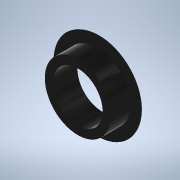
# Autodesk Inventor part: 08-02-01-010_buttonSide
Saved by Autodesk Inventor 2020 (Build 240168000, 168)
## iProperties
Created: 2021-08-25
Part Number: 08-02-01-010_buttonSide
Material: ABS-Kunststoff(1)
Document SubType Name: Modeling
Designer: Eric
Density: 1.06 g/cm^3
Appearance: Glatt - Weiß(1)
Author: Eric
Autodesk Inventor part; units mm, degrees
ref_plane "YZ Plane" through (0, 0, 0) normal (1, 0, 0) x (0, 1, 0)
ref_plane "XZ Plane" through (0, 0, 0) normal (0, 1, 0) x (-1, 0, 0)
ref_plane "XY Plane" through (0, 0, 0) normal (0, 0, 1) x (1, 0, 0)
sketch "Skizze1" plane through (0, 0, 0) normal (0, 1, 0) x (-1, 0, 0)
  line L0 (6.1, 0) -> (8.6, 0.5101)
  arc A0 (8.6, 0.5101) -> (9, 1) centre (8.5, 1) ccw
  line L1 (9, 1) -> (6.8, 1)
  line L2 (6.8, 1) -> (6.8, 5)
  line L3 (6.8, 5) -> (5.1, 5)
  line L4 (5.1, 5) -> (5.1, 0)
  line L5 (5.1, 0) -> (6.1, 0)
  line L6 (0, 0) -> (0, 11) construction
  dimension "d0" = 6.8
  dimension "d1" = 5.1
  dimension "d2" = 1
  dimension "d3" = 9
  dimension "d4" = 1
  dimension "d6" = 4
  dimension "d8" = 0.5
  constraints: 15 end point, 3 perpendicular, 2 point on circle, 1 centre point, 1 horizontal, 1 horizontal alignment, 1 line through centre, 1 tangent, 1 vertical
  measures "d0" distance from line of L6.start L2
  measures "d1" distance of L6.start L4.end
  measures "d2" distance of L4.end L0.start
  measures "d3" horizontal distance of L6.start L1.start
  measures "d4" distance between parallel lines of L5 L1
  measures "d6" distance between parallel lines of L3 L1
  measures "d8" radius of A0
revolve "Umdrehung1" add sketch "Skizze1" angle 360 about axis through (0, 0, 0) along (0, 0, 1)
